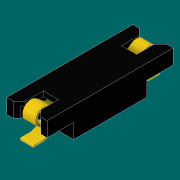
# Autodesk Inventor part: 788640001
Saved by Autodesk Inventor 2016 (Build 200138000, 138)
## iProperties
Created: 2015-10-16
Part Number: 788640001
Material: ABS Plastic
Document SubType Name: Modeling
Designer: Sawaiz
Density: 1.06 g/cm^3
Appearance: Smooth - Black
Author: Sawaiz
Autodesk Inventor part; units mm, degrees
ref_plane "YZ Plane" through (0, 0, 0) normal (1, 0, 0) x (0, 1, 0)
ref_plane "XZ Plane" through (0, 0, 0) normal (0, 1, 0) x (-1, 0, 0)
ref_plane "XY Plane" through (0, 0, 0) normal (0, 0, 1) x (1, 0, 0)
sketch "Sketch1" plane through (0, 0, 0) normal (0, 0, 1) x (1, 0, 0)
  line L0 (2.5, -0.8) -> (-2.5, -0.8)
  line L1 (-2.5, -0.8) -> (-2.5, 0.8)
  line L2 (-2.5, 0.8) -> (2.5, 0.8)
  line L3 (2.5, 0.8) -> (2.5, -0.8)
  line L4 (2.5, -0.8) -> (-2.5, 0.8) construction
  line L5 (-2.5, -0.8) -> (2.5, 0.8) construction
  line L6 (-2.5, -0.3) -> (-1.55, -0.3)
  line L7 (-1.55, -0.3) -> (-1.55, 0.3)
  line L8 (-1.55, 0.3) -> (-2.5, 0.3)
  line L9 (-2.5, 0.3) -> (-2.5, -0.3)
  line L10 (0, -0.8) -> (0, 0.8)
  line L11 (2.5, -0.3) -> (1.55, -0.3)
  line L12 (1.55, -0.3) -> (1.55, 0.3)
  line L13 (1.55, 0.3) -> (2.5, 0.3)
  line L14 (2.5, 0.3) -> (2.5, -0.3)
  point P0 (0, 0)
  point P1 (-2.5, 0)
  point P2 (2.5, 0)
  dimension "d0" = 5
  dimension "d1" = 1.6
  dimension "d2" = 0.95
  dimension "d3" = 0.6
  constraints: 30 end point, 6 midpoint, 5 symmetric about line, 4 parallel, 2 horizontal, 2 perpendicular, 1 point on line
  measures "d0" distance of L1.end L2.end
  measures "d1" distance of L0.end L1.end
  measures "d2" distance of L8.end L7.end
  measures "d3" distance between parallel lines of L8 L6
extrude "Extrusion1" add sketch "Sketch1" along normal blind 1.17 contours L0 L10 L2 L3 L13 L12 L11 | L0 L1 L6 L7 L8 L2 L10
sketch "Sketch2" plane through (-2.5, 0.8, 0) normal (0, 1, 0) x (1, 0, 0)
  line L0 (5, 0) -> (0, 0) projected
  line L1 (0, 0) -> (0, -1.17) projected
  line L2 (5, -1.17) -> (0, -1.17) projected
  line L3 (5, 0) -> (5, -1.17) projected
  line L4 (5, 0) -> (3.95, 0)
  line L5 (3.95, 0) -> (3.95, -0.585)
  line L6 (3.95, -0.585) -> (5, -0.585)
  line L7 (5, -0.585) -> (5, 0)
  line L8 (2.5, 0) -> (2.5, -1.17)
  line L9 (0, 0) -> (1.05, 0)
  line L10 (1.05, 0) -> (1.05, -0.585)
  line L11 (1.05, -0.585) -> (0, -0.585)
  line L12 (0, -0.585) -> (0, 0)
  dimension "d6" = 0.585
  dimension "d7" = 2.9
  constraints: 18 end point, 3 symmetric about line, 2 parallel, 1 horizontal, 1 midpoint, 1 perpendicular
  measures "d6" distance of L4.end L5.end
  measures "d7" distance between parallel lines of L10 L5
extrude "Extrusion2" cut sketch "Sketch2" against normal through all contours L3 L6 L5 L0 | L10 L11 L1 L0
sketch "Sketch3" plane through (1.45, 0.8, 0.585) normal (1, 0, 0) x (0, 0, -1)
  line L0 (0.585, -1.6) -> (0, -1.6) projected
  line L1 (0.585, 0) -> (0.585, -1.6) projected
  line L2 (0, 0) -> (0.585, 0) projected
  line L3 (0, 0) -> (0, -1.6) projected
  line L4 (0, -1.6) -> (0, -1.1) projected
  line L5 (0, -1.1) -> (-0.585, -1.1) projected
  line L6 (-0.585, -1.6) -> (-0.585, -1.1) projected
  line L7 (0, -1.6) -> (-0.585, -1.6) projected
  line L8 (0, -1.1) -> (0, -0.5) projected
  line L9 (0, -0.5) -> (-0.585, -0.5) projected
  line L10 (-0.585, -1.1) -> (-0.585, -0.5) projected
  line L11 (0, -1.1) -> (-0.585, -1.1) projected
  line L12 (0, -0.5) -> (0, 0) projected
  line L13 (0, 0) -> (-0.585, 0) projected
  line L14 (-0.585, -0.5) -> (-0.585, 0) projected
  line L15 (-0.585, -0.5) -> (0, -0.5) projected
  line L16 (0.385, -1.2) -> (-0.385, -1.2)
  line L17 (-0.385, -1.2) -> (-0.385, -0.4)
  line L18 (-0.385, -0.4) -> (0.385, -0.4)
  line L19 (0.385, -0.4) -> (0.385, -1.2)
  point P0 (0.585, -0.8)
  dimension "d10" = 0.4
  dimension "d11" = 0.4
  dimension "d12" = 0.2
  dimension "d13" = 0.2
  constraints: 8 end point, 2 parallel, 1 horizontal, 1 perpendicular
  measures "d10" distance between parallel lines of L2 L18
  measures "d11" distance between parallel lines of L0 L16
  measures "d12" distance between parallel lines of L10 L17
  measures "d13" distance between parallel lines of L1 L19
extrude "Extrusion3" cut sketch "Sketch3" along normal through all both and the other way through all contours L16 L17 L5 L3 | L3 L18 L19 L16 | L5 L17 L9 L3 | L3 L9 L17 L18
sketch "Sketch4" plane through (0, 0, 0) normal (0, 1, 0) x (-1, 0, 0)
  line L0 (2.5, 0.97) -> (2.5, 0.585) projected
  line L1 (-2.5, 0.97) -> (2.5, 0.97) projected
  line L2 (-2.5, 0.585) -> (-2.5, 0.97) projected
  line L3 (-1.45, 0.585) -> (-2.5, 0.585) projected
  line L4 (-1.45, 0.2) -> (-1.45, 0.585) projected
  line L5 (1.45, 0.2) -> (-1.45, 0.2) projected
  line L6 (1.45, 0.585) -> (1.45, 0.2) projected
  line L7 (2.5, 0.585) -> (1.45, 0.585) projected
  line L8 (-0.1, 0.97) -> (0.1, 0.97)
  line L9 (0.1, 0.97) -> (0.1, 0.2)
  line L10 (0.1, 0.2) -> (-0.1, 0.2)
  line L11 (-0.1, 0.2) -> (-0.1, 0.97)
  point P0 (0, 0)
  point P1 (0, 0.97)
  dimension "d16" = 0.2
  constraints: 8 end point, 2 midpoint, 2 parallel, 2 point on line, 1 horizontal, 1 perpendicular
  measures "d16" distance between parallel lines of L11 L9
extrude "Extrusion4" add sketch "Sketch4" along normal mid plane 1.6 contours L9 L5 L11 L1
sketch "Sketch5" plane through (0, 0, 0) normal (0, 1, 0) x (-1, 0, 0)
  line L0 (-0.1, 0.2) -> (-0.1, 0.97) projected
  line L1 (-2.5, 0.97) -> (-0.1, 0.97) projected
  line L2 (-2.5, 0.585) -> (-2.5, 0.97) projected
  line L3 (-1.45, 0.585) -> (-2.5, 0.585) projected
  line L4 (-1.45, 0.2) -> (-1.45, 0.585) projected
  line L5 (-0.1, 0.2) -> (-1.45, 0.2) projected
  line L6 (-0.1, 0.2) -> (-1.45, 0.2) projected
  arc A0 (-0.485, 0.2) -> (-0.5332, 0.967) centre (-0.485, 0.585) ccw
  arc A1 (-0.537, 0.2845) -> (-0.5232, 0.8876) centre (-0.485, 0.585) ccw
  line L7 (-0.485, 0.2) -> (-1.45, 0.2)
  line L8 (-1.45, 0.2) -> (-2.1, -0.02)
  line L9 (-2.1, -0.02) -> (-2.5, -0.02)
  line L10 (-2.5, -0.02) -> (-2.5, 0.06)
  line L11 (-2.5, 0.06) -> (-2.1132, 0.06)
  line L12 (-2.1132, 0.06) -> (-1.45, 0.2845)
  line L13 (-1.45, 0.2845) -> (-0.537, 0.2845)
  line L14 (1.45, 0) -> (-1.45, 0) projected
  line L15 (-0.5332, 0.967) -> (-1.55, 0.8387)
  line L16 (-1.55, 0.8387) -> (-1.8877, 1.1007)
  line L17 (-0.5232, 0.8876) -> (-1.5729, 0.7552)
  line L18 (-1.5729, 0.7552) -> (-1.9367, 1.0375)
  arc A2 (-1.8877, 1.1007) -> (-2.2923, 0.5793) centre (-2.09, 0.84) ccw
  arc A3 (-1.9367, 1.0375) -> (-2.2433, 0.6425) centre (-2.09, 0.84) ccw
  line L19 (2.5, 1.17) -> (-2.5, 1.17) projected
  line L20 (-1.55, 0.97) -> (-1.55, 1.17) projected
  line L21 (-2.2923, 0.5793) -> (-1.7814, 0.1829)
  line L22 (-1.7814, 0.1829) -> (-1.3078, 0.3431)
  line L23 (-1.3078, 0.3431) -> (-1.3334, 0.4189)
  line L24 (-1.3334, 0.4189) -> (-1.7663, 0.2724)
  line L25 (-1.7663, 0.2724) -> (-2.2433, 0.6425)
  line L26 (-2.2923, 0.5793) -> (-2.2879, 0.585)
  line L27 (-0.1, 0.97) -> (-0.2128, 0.8572)
  point P0 (0, 0)
  point P1 (0, 1.17)
  dimension "d20" = 0.08
  dimension "d21" = 0.08
  dimension "d22" = 0.08
  dimension "d23" = 0.02
  dimension "d25" = 0.4
  dimension "d26" = 0.08
  dimension "d27" = 0.5
  dimension "d29" = 2.09
  dimension "d30" = 135
  dimension "d31" = 0
  dimension "d32" = 0.08
  dimension "d33" = 0.01
  dimension "d34" = 0.5
  constraints: 36 end point, 9 point on circle, 8 parallel, 8 tangent, 4 centre point, 4 point on line, 3 perpendicular, 2 coincident, 2 collinear, 1 midpoint
  measures "d20" radial gap between concentric circles of A0 A1
  measures "d21" distance between parallel lines of L11 L9
  measures "d22" distance between parallel lines of L8 L12
  measures "d23" distance between parallel lines of L9 L14
  measures "d25" distance of L8.end L9.end
  measures "d26" radial gap between concentric circles of A2 A3
  measures "d27" diameter of A3
  measures "d29" horizontal distance of A2.centre point (0, 1.17)
  measures "d30" angle of L16 L15
  measures "d31" distance from line of L20 L15.end
  measures "d32" distance between parallel lines of L24 L22
  measures "d33" distance between parallel lines of L22 L12
  measures "d34" distance from line of L21.end L23
extrude "Extrusion5" add sketch "Sketch5" along normal mid plane 0.5 separate body contours A0 L5 L4 L13 A1 L17 L18 L1 L16 L15 | L8 L9 L10 L11 L12 L4 | L22 L21 L26 L3 L25 L24 L4 | L4 L24 L23 L22 | L1 L18 A3 A2 L16 | A2 L3 L26 | A3 L25 L3 A2 L1
mirror "Mirror1" about plane through (0, 0, 0) normal (1, 0, 0) of "Extrusion5" bodies 2
sketch "Sketch6" plane through (0, 0, 1.17) normal (0, 0, 1) x (1, 0, 0)
  line L0 (2.5, -0.3) -> (1.55, -0.3) projected
  line L1 (1.55, -0.3) -> (1.55, 0.3) projected
  line L2 (1.55, 0.3) -> (2.5, 0.3) projected
  line L3 (2.5, 0.3) -> (2.5, 0.8) projected
  line L4 (2.5, 0.8) -> (-2.5, 0.8) projected
  line L5 (-2.5, 0.8) -> (-2.5, 0.3) projected
  line L6 (-2.5, 0.3) -> (-1.55, 0.3) projected
  line L7 (-1.55, 0.3) -> (-1.55, -0.3) projected
  line L8 (-1.55, -0.3) -> (-2.5, -0.3) projected
  line L9 (-2.5, -0.3) -> (-2.5, -0.8) projected
  line L10 (-2.5, -0.8) -> (2.5, -0.8) projected
  line L11 (2.5, -0.8) -> (2.5, -0.3) projected
  line L12 (2.5, -0.55) -> (2.25, -0.3)
  line L13 (2.5, -0.3) -> (1.55, -0.3) projected
  line L14 (2.5, 0.55) -> (2.25, 0.3)
  line L15 (-2.5, -0.3) -> (-2.5, -0.8) projected
  line L16 (-2.5, -0.55) -> (-2.25, -0.3)
  line L17 (-1.55, -0.3) -> (-2.5, -0.3) projected
  line L18 (-2.5, 0.8) -> (-2.5, 0.3) projected
  line L19 (-2.5, 0.55) -> (-2.25, 0.3)
  line L20 (-2.5, 0.3) -> (-1.55, 0.3) projected
  point P0 (0, 0)
  dimension "d37" = 45
  constraints: 8 end point, 4 midpoint, 4 point on line, 3 perpendicular
  measures "d37" angle of L5 L19
extrude "Extrusion6" cut sketch "Sketch6" against normal through all contours L11 L12 L0 | L14 L3 L2 | L9 L8 L16 | L19 L6 L5 bodies 1
body "Solid1"
body "Solid2"
